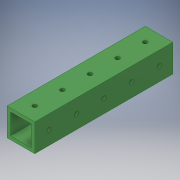
# Autodesk Inventor part: Kermit Frame 12
Saved by Autodesk Inventor 2018.2 (Build 222227000, 227)
## iProperties
Created: 2018-02-06
Part Number: Kermit Frame 12
Material: Generic
Document SubType Name: Modeling
Designer: lopez.xavier
Density: 1 g/cm^3
Appearance: Smooth - Dark Forest Green
Author: lopez.xavier
Autodesk Inventor part; units mm, degrees
ref_plane "YZ Plane" through (0, 0, 0) normal (1, 0, 0) x (0, 1, 0)
ref_plane "XZ Plane" through (0, 0, 0) normal (0, 1, 0) x (-1, 0, 0)
ref_plane "XY Plane" through (0, 0, 0) normal (0, 0, 1) x (1, 0, 0)
sketch "Sketch1" plane through (0, 0, 0) normal (0, 0, 1) x (1, 0, 0)
  line L0 (0, 0) -> (25.4, 0)
  line L1 (25.4, 0) -> (25.4, 25.4)
  line L2 (25.4, 25.4) -> (0, 25.4)
  line L3 (0, 25.4) -> (0, 0)
  dimension "d0" = 25.4
  dimension "d1" = 25.4
  constraints: 8 end point, 2 parallel, 1 horizontal, 1 perpendicular
  measures "d0" distance of L2.end L1.end
  measures "d1" distance of L1.end L0.end
extrude "Extrusion1" add sketch "Sketch1" along normal blind 127
shell "Shell1" thickness 3.175 removed faces 2 at (8.4667, 16.9333, 0) at (8.4667, 16.9333, 127)
sketch "Sketch2" plane through (0, 25.4, 0) normal (0, 1, 0) x (1, 0, 0)
  circle A0 centre (12.7, -12.7) radius 1.9685
  line L0 (0, 0) -> (0, -127) projected
  line L1 (25.4, 0) -> (0, 0) projected
  circle A1 centre (12.7, -38.1) radius 1.9685
  circle A2 centre (12.7, -63.5) radius 1.9685
  circle A3 centre (12.7, -88.9) radius 1.9685
  circle A4 centre (12.7, -114.3) radius 1.9685
  dimension "d5" = 3.937
  dimension "d6" = 12.7
  dimension "d7" = 12.7
  dimension "d10" = 25.4
  constraints: 5 centre point, 1 vertical, 8 other
  measures "d5" diameter of A0
  measures "d6" distance from line of L0 A0.centre
  measures "d7" distance from line of L1 A0.centre
  measures "d10" distance of A0.centre A1.centre
extrude "Extrusion2" cut sketch "Sketch2" against normal blind 127
sketch "Sketch3" plane through (25.4, 0, 0) normal (1, 0, 0) x (0, 0, -1)
  circle A0 centre (-12.7, 12.7) radius 1.9685
  line L0 (0, 25.4) -> (-127, 25.4) projected
  line L1 (0, 0) -> (0, 25.4) projected
  circle A1 centre (-38.1, 12.7) radius 1.9685
  circle A2 centre (-63.5, 12.7) radius 1.9685
  circle A3 centre (-88.9, 12.7) radius 1.9685
  circle A4 centre (-114.3, 12.7) radius 1.9685
  dimension "d17" = 3.937
  dimension "d18" = 12.7
  dimension "d19" = 12.7
  dimension "d22" = 25.4
  constraints: 5 centre point, 1 horizontal, 8 other
  measures "d17" diameter of A0
  measures "d18" distance from line of L0 A0.centre
  measures "d19" distance from line of L1 A0.centre
  measures "d22" distance of A0.centre A1.centre
extrude "Extrusion3" cut sketch "Sketch3" against normal blind 127
body "Solid1"
